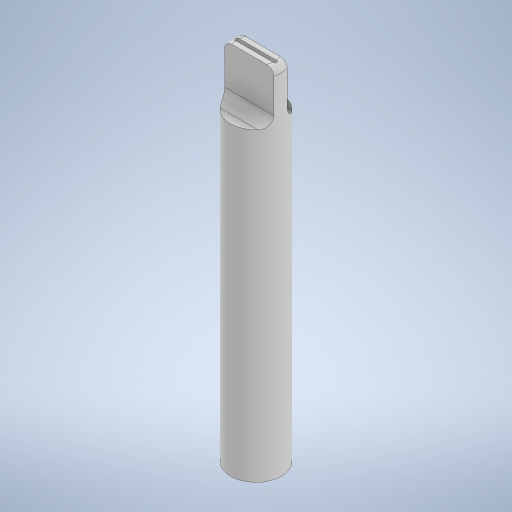
# Autodesk Inventor part: PUFIK_2
Saved by Autodesk Inventor 2023 (Build 270158000, 158)
## iProperties
Created: 2024-04-21
Part Number: PUFIK_2
Material: Generic
Document SubType Name: Modeling
Designer: VRACOVSKÝ
Density: 1 g/cm^3
Appearance: Default
Author: vraco
Autodesk Inventor part; units mm, degrees
ref_plane "YZ Plane" through (0, 0, 0) normal (1, 0, 0) x (0, 1, 0)
ref_plane "XZ Plane" through (0, 0, 0) normal (0, 1, 0) x (-1, 0, 0)
ref_plane "XY Plane" through (0, 0, 0) normal (0, 0, 1) x (1, 0, 0)
sketch "Sketch1" plane through (0, 0, 0) normal (0, 1, 0) x (-1, 0, 0)
  line L0 (0, -10.5) -> (0, 10.5) projected
  line L1 (-10.5, 0) -> (10.5, 0) projected
  circle A0 centre (0, 0) radius 7.5
  dimension "d0" = 15
  constraints: 1 centre point, 1 coincident
  measures "d0" diameter of A0
extrude "Extrusion1" add sketch "Sketch1" along normal blind 90
sketch "Sketch2" plane through (0, 90, 0) normal (0, 1, 0) x (1, 0, 0)
  line L0 (10.5, 0) -> (-10.5, 0) projected
  line L1 (0, 10.5) -> (0, -10.5) projected
  line L2 (-7.2284, 2) -> (7.2284, 2)
  line L3 (-7.2284, -2) -> (7.2284, -2)
  circle A0 centre (0, 0) radius 7.5 projected
  arc A1 (7.2284, -2) -> (7.2284, 2) centre (0, 0) ccw
  arc A2 (-7.2284, 2) -> (-7.2284, -2) centre (0, 0) ccw
  point P0 (7.2284, -2)
  dimension "d3" = 4
  dimension "d4" = 15
  dimension "d5" = 4
  constraints: 4 end point, 4 point on circle, 2 centre point, 2 horizontal, 1 coincident, 1 other
  measures "d3" distance between parallel lines of L2 L3
  measures "d4" diameter of A0
  measures "d5" distance of L2.end L3.end
extrude "Extrusion2" add sketch "Sketch2" along normal blind 15 contours A0 L3 L1 L0 | L0 L1 L2 A0 | L1 L3 A0 L0 | L0 A0 L2 L1
fillet "Fillet1" radius 3 2 edges at (0, 90, 2) (0, 90, -2)
sketch "Sketch3" plane through (0, 105, 0) normal (0, 1, 0) x (1, 0, 0)
  line L0 (-7.2284, -2) -> (7.2284, -2) projected
  line L1 (7.2284, 2) -> (-7.2284, 2) projected
  arc A0 (7.2284, -2) -> (7.2284, 2) centre (0, 0) ccw projected
  arc A1 (-7.2284, 2) -> (-7.2284, -2) centre (0, 0) ccw projected
  line L2 (-5.9791, 0.5) -> (5.9791, 0.5)
  arc A2 (5.9791, -0.5) -> (5.9791, 0.5) centre (0, 0) ccw
  line L3 (5.9791, -0.5) -> (-5.9791, -0.5)
  arc A3 (-5.9791, 0.5) -> (-5.9791, -0.5) centre (0, 0) ccw
  dimension "d9" = 1.5
  constraints: 4 end point, 4 point on circle, 2 centre point, 3 other
  measures "d9" distance between parallel lines of L1 L2
extrude "Extrusion3" cut sketch "Sketch3" against normal blind 15 contours L2 A2 L3 A3
fillet "Fillet2" radius 2 2 edges at (7.5, 105, 0) (-7.5, 105, 0)
body "Solid1"
